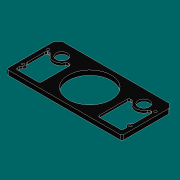
# Autodesk Inventor part: 胴体_メインフレーム_1_2
Saved by Autodesk Inventor 2016 (Build 200138000, 138)
## iProperties
Created: 2016-05-05
Part Number: 胴体_メインフレーム_1_2
Material: アセタール樹脂、黒
Document SubType Name: Modeling
Designer: hiroaki
Density: 1.425 g/cm^3
Appearance: 滑らか - 黒
Mass: 18.1472 g
Surface Area: 107.175 cm^2
Volume: 12.7348 cm^3
Author: hiroaki
Autodesk Inventor part; units mm, degrees
ref_plane "YZ Plane" through (0, 0, 0) normal (1, 0, 0) x (0, 1, 0)
ref_plane "XZ Plane" through (0, 0, 0) normal (0, 1, 0) x (-1, 0, 0)
ref_plane "XY Plane" through (0, 0, 0) normal (0, 0, 1) x (1, 0, 0)
derived "胴体_基礎_1_1.ipt"
sketch "スケッチ1" plane through (0, 0, 0) normal (0, 0, 1) x (1, 0, 0)
  circle A0 centre (44, 0) radius 10.5 construction
  line L0 (0, 0) -> (0, 13.5711) construction
  line L1 (0, 0) -> (44, 0) construction
  line L2 (30.5, -1) -> (57.5, -1) construction
  line L3 (57.5, -1) -> (57.5, -28) construction
  line L4 (57.5, -28) -> (30.5, -28) construction
  line L5 (30.5, -28) -> (30.5, -1) construction
  circle A1 centre (30.5, -1) radius 1.35
  circle A2 centre (57.5, -1) radius 1.35
  circle A3 centre (30.5, -28) radius 1.35
  circle A4 centre (57.5, -28) radius 1.35
  line L6 (28, 0) -> (28, -39.5) construction
  line L7 (28, -39.5) -> (60, -39.5) construction
  line L8 (60, -39.5) -> (60, 0) construction
  line L9 (44, 0) -> (44, -1) construction
  arc A5 (33.417, 12) -> (28, 0) centre (44, 0) ccw construction
  line L10 (33.417, 12) -> (54.583, 12) construction
  arc A6 (60, 0) -> (54.583, 12) centre (44, 0) ccw construction
  circle A7 centre (44, 0) radius 11
  line L11 (56.5, 21.6506) -> (8, -62.3538) construction
  line L12 (31.8157, -76.1038) -> (-15.8157, -48.6038) construction
  line L13 (-15.8157, -48.6038) -> (32.6843, 35.4006) construction
  line L14 (32.6843, 35.4006) -> (80.3157, 7.9006) construction
  line L15 (80.3157, 7.9006) -> (31.8157, -76.1038) construction
  line L16 (-71.5, 25) -> (-16.5, 25) construction
  line L17 (-16.5, 25) -> (-16.5, -72) construction
  line L18 (-16.5, -72) -> (-71.5, -72) construction
  line L19 (-71.5, -72) -> (-71.5, 25) construction
  line L20 (-44, 25) -> (-44, -72) construction
  line L21 (-71.5, 0) -> (-16.5, 0) construction
  line L22 (-52.5, -44.5) -> (52.5, -44.5) construction
  line L23 (52.5, -44.5) -> (52.5, -78) construction
  line L24 (52.5, -78) -> (-52.5, -78) construction
  line L25 (-52.5, -78) -> (-52.5, -44.5) construction
  line L26 (-44.5, -5) -> (44.5, -5) construction
  line L27 (44.5, -5) -> (44.5, -65) construction
  line L28 (44.5, -65) -> (-44.5, -65) construction
  line L29 (-44.5, -65) -> (-44.5, -5) construction
  circle A8 centre (44, 24.25) radius 1.2
  circle A9 centre (19.75, 0) radius 1.2
  circle A10 centre (44, -24.25) radius 1.2
  circle A11 centre (68.25, 0) radius 1.2
  line L30 (-45.0355, 26.75) -> (45.0355, 26.75) construction
  circle A12 centre (44, 24.25) radius 2.5 construction
  line L31 (46, 25.4047) -> (46, 23.0953) construction
  line L32 (46, 23.0953) -> (44, 21.9406) construction
  line L33 (44, 21.9406) -> (42, 23.0953) construction
  line L34 (42, 23.0953) -> (42, 25.4047) construction
  line L35 (42, 25.4047) -> (44, 26.5594) construction
  line L36 (44, 26.5594) -> (46, 25.4047) construction
  line L37 (70.75, 1.0355) -> (70.75, -31.2817) construction
  line L38 (-70.75, -31.2817) -> (-70.75, 1.0355) construction
  circle A13 centre (68.25, 0) radius 2.5 construction
  circle A14 centre (-44, 24.25) radius 1.2
  circle A15 centre (-19.75, 0) radius 1.2
  circle A16 centre (-30.5, -1) radius 1.35
  circle A17 centre (-44, 0) radius 11
  circle A18 centre (-57.5, -1) radius 1.35
  circle A19 centre (-44, -24.25) radius 1.2
  circle A20 centre (-30.5, -28) radius 1.35
  circle A21 centre (-57.5, -28) radius 1.35
  circle A22 centre (-68.25, 0) radius 1.2
  line L39 (-45.0355, 26.75) -> (-70.75, 1.0355) construction
  line L40 (45.0355, 26.75) -> (70.75, 1.0355) construction
  line L41 (70.75, 1.0355) -> (70.75, -1.0355)
  line L42 (-70.75, 1.0355) -> (-70.75, -1.0355) construction
  circle A23 centre (44, 0) radius 6.05
  circle A24 centre (-44, 0) radius 6.05
  line L43 (-70.75, -1.0355) -> (-62, -9.7855) construction
  line L44 (-62, -9.7855) -> (-62, -33) construction
  line L45 (-62, -33) -> (62, -33) construction
  line L46 (62, -33) -> (62, -9.7855) construction
  line L47 (62, -9.7855) -> (70.75, -1.0355) construction
  line L48 (57.7855, 14) -> (-57.7855, 14)
  line L49 (-57.7855, 14) -> (-62, 9.7855)
  line L50 (-62, 9.7855) -> (-62, -41.5)
  line L51 (-62, -41.5) -> (62, -41.5)
  line L52 (62, -41.5) -> (62, 9.7855)
  line L53 (62, 9.7855) -> (57.7855, 14)
  line L54 (21.5, -5) -> (26.5, -5) construction
  line L55 (19.75, 0) -> (28, 0) construction
  circle A25 centre (22.5, -28) radius 1.55 construction
  circle A26 centre (22.5, 21.75) radius 1.55 construction
  circle A27 centre (-22.5, 21.75) radius 1.55 construction
  circle A28 centre (-22.5, -28) radius 1.55 construction
  circle A29 centre (19.75, 0) radius 2 construction
  circle A30 centre (22.5, 21.75) radius 3 construction
  circle A31 centre (-22.5, 21.75) radius 1.2
  circle A32 centre (-22.5, -28) radius 1.2
  circle A33 centre (22.5, 21.75) radius 1.2
  circle A34 centre (22.5, -28) radius 1.2
  line L56 (-25.05, 15.75) -> (-19.95, 15.75) construction
  line L57 (-19.95, 15.75) -> (-19.95, 5.75) construction
  line L58 (-19.95, 5.75) -> (-25.05, 5.75) construction
  line L59 (-25.05, 5.75) -> (-25.05, 15.75) construction
  line L60 (-25.05, -4) -> (-19.95, -4) construction
  line L61 (-19.95, -4) -> (-19.95, -22) construction
  line L62 (-19.95, -22) -> (-25.05, -22) construction
  line L63 (-25.05, -22) -> (-25.05, -4) construction
  circle A35 centre (-19.75, 0) radius 2.5 construction
  line L64 (-19.9, 15.8) -> (-25.1, 15.8)
  line L65 (-25.1, 15.8) -> (-25.1, 5.7)
  line L66 (-25.1, 5.7) -> (-19.9, 5.7)
  line L67 (-19.9, 5.7) -> (-19.9, 15.8)
  circle A36 centre (-25.1, 14.75) radius 1.05
  circle A37 centre (-19.9, 14.75) radius 1.05
  circle A38 centre (-19.9, 6.75) radius 1.05
  circle A39 centre (-25.1, 6.75) radius 1.05
  line L68 (-19.9, -3.95) -> (-25.1, -3.95)
  line L69 (-25.1, -3.95) -> (-25.1, -22.05)
  line L70 (-25.1, -22.05) -> (-19.9, -22.05)
  line L71 (-19.9, -22.05) -> (-19.9, -3.95)
  circle A40 centre (-25.1, -5) radius 1.05
  circle A41 centre (-19.9, -5) radius 1.05
  circle A42 centre (-25.1, -21) radius 1.05
  circle A43 centre (-19.9, -21) radius 1.05
  line L72 (25.1, 15.8) -> (25.1, 5.7)
  circle A44 centre (25.1, 14.75) radius 1.05
  line L73 (19.9, 15.8) -> (25.1, 15.8)
  circle A45 centre (19.9, 14.75) radius 1.05
  line L74 (19.9, 5.7) -> (19.9, 15.8)
  circle A46 centre (25.1, 6.75) radius 1.05
  circle A47 centre (19.9, 6.75) radius 1.05
  line L75 (25.1, 5.7) -> (19.9, 5.7)
  circle A48 centre (25.1, -5) radius 1.05
  circle A49 centre (19.9, -5) radius 1.05
  line L76 (19.9, -3.95) -> (25.1, -3.95)
  line L77 (19.9, -22.05) -> (19.9, -3.95)
  line L78 (25.1, -3.95) -> (25.1, -22.05)
  circle A50 centre (25.1, -21) radius 1.05
  circle A51 centre (19.9, -21) radius 1.05
  line L79 (25.1, -22.05) -> (19.9, -22.05)
  circle A52 centre (44, 0) radius 21.9406 construction
  point P0 (0, -44.5)
  point P1 (-44.5, -35)
  point P2 (0, -5)
  point P3 (-22.5, 15.75)
  point P4 (-22.5, -4)
  point P5 (-22.5, 5.75)
  dimension "d60" = 12.1
  dimension "d61" = 2
  dimension "d64" = 2.4
  dimension "d66" = 14
  measures "d60" diameter of A23
  measures "d61" distance between parallel lines of L51 L7
  measures "d64" diameter of A31
  measures "d66" distance from line of L48 A17.centre
extrude "押し出し1" add sketch "スケッチ1" along normal blind 2.5 contours A1 | A3 | A7 | A9 | A10 | A15 | A16 | A17 | A19 | A20 | L53 L52 L51 L50 L49 L48 A36 L65 A39 L66 A38 L67 A37 A45 L74 A47 L75 A46 L72 A44 | A44 L72 L48 | L72 A44 L48 | L72 A46 L75 A47 L74 A45 L48 A44 | A46 L72 | L72 A46 | A45 L74 L48 | L74 A45 L48 | A47 L74 | L74 A47 | A37 L67 L48 | L48 L65 A36 | L67 A37 L48 | L67 A38 L66 A39 L65 A36 L48 A37 | L48 A36 L65 | A38 L67 | L67 A38 | A39 L65 | L65 A39 | A32 | A34 | A41 L71 A43 L70 A42 L69 A40 L68 | A41 L71 | L71 A41 | A40 L69 | L69 A40 | A43 L71 | L71 A43 | A42 L69 | L69 A42 | A48 L78 | L78 A48 | A48 L78 A50 L79 A51 L77 A49 L76 | L77 A49 | A49 L77 | A50 L78 | L78 A50 | A51 L77 | L77 A51 picked at (25.5372, 13.9575) picked at (24.6628, 13.9575) picked at (20.3372, 13.9575) picked at (19.4628, 13.9575) picked at (-19.4628, 13.9575) picked at (-25.5372, 13.9575) picked at (-20.3372, 13.9575) picked at (-24.6628, 13.9575)
mirror "ミラー1" about plane through (0, -14.1578, 0) normal (0, 0, -1) of "押し出し1"
sketch "スケッチ4" plane through (62, -41.5, -2.5) normal (0, 0, -1) x (-1, 0, 0)
  circle A0 centre (106, 41.5) radius 5.05
  circle A1 centre (4.5, 13.5) radius 1.35 projected
  circle A2 centre (4.5, 40.5) radius 1.35 projected
  circle A3 centre (119.5, 13.5) radius 1.35 projected
  circle A4 centre (119.5, 40.5) radius 1.35 projected
  line L0 (7.417, 53.5) -> (28.583, 53.5) construction
  line L1 (2, 41.5) -> (2, 2) construction
  line L2 (2, 2) -> (34, 2) construction
  line L3 (34, 2) -> (34, 41.5) construction
  arc A5 (7.417, 53.5) -> (2, 41.5) centre (18, 41.5) ccw construction
  arc A6 (34, 41.5) -> (28.583, 53.5) centre (18, 41.5) ccw construction
  line L4 (1.95, 1.95) -> (1.95, 41.5)
  arc A7 (7.3981, 53.55) -> (1.95, 41.5) centre (18, 41.5) ccw
  line L5 (7.3981, 53.55) -> (28.6019, 53.55)
  arc A8 (34.05, 41.5) -> (28.6019, 53.55) centre (18, 41.5) ccw
  line L6 (34.05, 41.5) -> (34.05, 1.95)
  line L7 (34.05, 1.95) -> (1.95, 1.95)
  circle A9 centre (3.3996, 3.3996) radius 2.05
  circle A10 centre (32.6004, 3.3996) radius 2.05
  circle A11 centre (27.7355, 51.6921) radius 2.05
  circle A12 centre (8.2645, 51.6921) radius 2.05
  line L8 (3.3996, 3.3996) -> (1.95, 1.95) construction
  line L9 (8.2645, 51.6921) -> (7.3981, 53.55) construction
  line L10 (62, 41.5) -> (62, 0) construction
  line L11 (122.05, 1.95) -> (122.05, 41.5)
  arc A13 (122.05, 41.5) -> (116.6019, 53.55) centre (106, 41.5) ccw
  line L12 (116.6019, 53.55) -> (95.3981, 53.55)
  arc A14 (95.3981, 53.55) -> (89.95, 41.5) centre (106, 41.5) ccw
  line L13 (89.95, 41.5) -> (89.95, 1.95)
  line L14 (89.95, 1.95) -> (122.05, 1.95)
  circle A15 centre (120.6004, 3.3996) radius 2.05
  circle A16 centre (91.3996, 3.3996) radius 2.05
  circle A17 centre (96.2645, 51.6921) radius 2.05
  circle A18 centre (115.7355, 51.6921) radius 2.05
  circle A19 centre (18, 41.5) radius 5.05
  circle A20 centre (106, 41.5) radius 5.05
  line L15 (124, 0) -> (0, 0) projected
  line L16 (18, 41.5) -> (18, 2) construction
  circle A21 centre (18, 41.5) radius 6.05 projected
  point P0 (18, 53.5)
  point P1 (62, 0)
  dimension "d56" = 4.1
  dimension "d52" = 16
  dimension "d53" = 51.5
  dimension "d54" = 0.05
  dimension "d55" = 45
  dimension "d57" = 65
  dimension "d62" = 10.1
  dimension "d63" = 12
  constraints: 32 end point, 16 symmetric about line, 12 point on circle, 9 centre point, 6 coincident, 6 vertical, 5 perpendicular, 4 midpoint, 2 tangent, 1 equal radius, 1 horizontal, 32 other
  measures "d52" radius of A5
  measures "d53" distance between parallel lines of L2 L0
  measures "d54" distance between parallel lines of L4 L1
  measures "d55" angle of L1 L8
  measures "d57" angle of L0 L9
  measures "d62" diameter of A19
  measures "d63" distance from line of A5.centre L0
extrude "押し出し2" cut sketch "スケッチ4" against normal blind 2.5 contours A9 L4 | L4 A9 L7 | L7 A9 | L4 A7 A12 L5 A11 A8 L6 A10 L7 A9 | A10 L6 L7 | L7 A10 | A12 A7 | A7 L5 A12 | L6 A10 | A12 L5 | A11 L5 A8 | A8 A11 | A11 L5 | L14 A15 L11 | A15 L14 | L11 A15 | A15 L14 A16 L13 A14 A17 L12 A18 A13 L11 | A16 L14 | L14 L13 A16 | A18 L12 A13 | A13 A18 | A16 L13 | L12 A18 | A17 A14 L12 | L12 A17 | A17 A14 | A19 | A21
sketch "スケッチ6" plane through (62, -41.5, -2.5) normal (0, 0, -1) x (-1, 0, 0)
  line L0 (34.05, 41.5) -> (34.05, 4.8491) construction
  line L1 (4.2145, 55.5) -> (119.7855, 55.5) projected
  circle A0 centre (62, 27.55) radius 27.95 construction
  circle A1 centre (62, 27.55) radius 22.95
  line L2 (31.1509, 1.95) -> (4.8491, 1.95) construction
  line L3 (1.95, 4.8491) -> (1.95, 41.5) construction
  arc A2 (6.4482, 52.6426) -> (1.95, 41.5) centre (18, 41.5) ccw construction
  line L4 (4.95, 37.6858) -> (4.95, 16.3142)
  line L5 (4.95, 10.6858) -> (4.95, 4.95)
  line L6 (4.95, 4.95) -> (31.05, 4.95)
  line L7 (31.05, 4.95) -> (31.05, 38.5)
  line L8 (6.5304, 38.5) -> (9.5147, 38.5)
  line L9 (31.05, 38.5) -> (26.4853, 38.5)
  arc A3 (9.5147, 38.5) -> (26.4853, 38.5) centre (18, 41.5) ccw
  arc A4 (4.95, 37.6858) -> (6.5304, 38.5) centre (4.5, 40.5) ccw
  circle A5 centre (4.5, 40.5) radius 1.35 construction
  circle A6 centre (4.5, 40.5) radius 1.35 construction
  arc A7 (4.95, 10.6858) -> (4.95, 16.3142) centre (4.5, 13.5) ccw
  circle A8 centre (4.5, 13.5) radius 1.35 construction
  circle A9 centre (4.5, 13.5) radius 1.35 construction
  line L10 (62, 41.5) -> (62, 27.55) construction
  line L11 (119.05, 37.6858) -> (119.05, 16.3142)
  line L12 (119.05, 10.6858) -> (119.05, 4.95)
  line L13 (119.05, 4.95) -> (92.95, 4.95)
  line L14 (92.95, 4.95) -> (92.95, 38.5)
  line L15 (117.4696, 38.5) -> (114.4853, 38.5)
  line L16 (92.95, 38.5) -> (97.5147, 38.5)
  arc A10 (97.5147, 38.5) -> (114.4853, 38.5) centre (106, 41.5) ccw
  arc A11 (117.4696, 38.5) -> (119.05, 37.6858) centre (119.5, 40.5) ccw
  arc A12 (119.05, 16.3142) -> (119.05, 10.6858) centre (119.5, 13.5) ccw
  arc A13 (1.95, 4.8491) -> (4.8491, 1.95) centre (3.3996, 3.3996) ccw construction
  arc A14 (9.1308, 53.55) -> (6.4482, 52.6426) centre (8.2645, 51.6921) ccw construction
  line L17 (9.1308, 53.55) -> (26.8692, 53.55) construction
  arc A15 (29.5518, 52.6426) -> (26.8692, 53.55) centre (27.7355, 51.6921) ccw construction
  arc A16 (34.05, 41.5) -> (29.5518, 52.6426) centre (18, 41.5) ccw construction
  arc A17 (31.1509, 1.95) -> (34.05, 4.8491) centre (32.6004, 3.3996) ccw construction
  line L18 (124, 0) -> (0, 0) projected
  line L19 (26.8803, 53.5) -> (9.1197, 53.5) construction
  arc A18 (9.1197, 53.5) -> (6.4892, 52.6131) centre (8.2645, 51.6921) ccw construction
  arc A19 (6.4892, 52.6131) -> (2, 41.5) centre (18, 41.5) ccw construction
  line L20 (2, 41.5) -> (2, 4.8283) construction
  arc A20 (2, 4.8283) -> (4.8283, 2) centre (3.3996, 3.3996) ccw construction
  line L21 (4.8283, 2) -> (31.1717, 2) construction
  arc A21 (31.1717, 2) -> (34, 4.8283) centre (32.6004, 3.3996) ccw construction
  line L22 (34, 4.8283) -> (34, 41.5) construction
  arc A22 (34, 41.5) -> (29.5108, 52.6131) centre (18, 41.5) ccw construction
  arc A23 (29.5108, 52.6131) -> (26.8803, 53.5) centre (27.7355, 51.6921) ccw construction
  line L23 (35.3205, 51.5) -> (47.5917, 51.5)
  arc A24 (37.9966, 41.8692) -> (35.3205, 51.5) centre (18, 41.5) ccw
  arc A25 (47.5917, 51.5) -> (37.9966, 41.8692) centre (62, 27.55) ccw
  line L24 (38, 13.2251) -> (38, 4)
  line L25 (38, 4) -> (46.9468, 4)
  arc A26 (38, 13.2251) -> (46.9468, 4) centre (62, 27.55) ccw
  line L26 (88.6795, 51.5) -> (76.4083, 51.5)
  arc A27 (88.6795, 51.5) -> (86.0034, 41.8692) centre (106, 41.5) ccw
  arc A28 (86.0034, 41.8692) -> (76.4083, 51.5) centre (62, 27.55) ccw
  line L27 (86, 13.2251) -> (86, 4)
  line L28 (86, 4) -> (77.0532, 4)
  arc A29 (77.0532, 4) -> (86, 13.2251) centre (62, 27.55) ccw
  dimension "d74" = 5
  dimension "d77" = 9
  dimension "d78" = 1.5
  dimension "d79" = 2
  dimension "d80" = 3
  dimension "d81" = 3
  dimension "d82" = 3
  dimension "d85" = 0.05
  dimension "d89" = 4
  dimension "d90" = 4
  dimension "d91" = 4
  dimension "d92" = 4
  constraints: 46 end point, 36 point on circle, 22 centre point, 19 symmetric about line, 8 coincident, 6 tangent, 4 horizontal, 4 vertical, 2 perpendicular, 2 vertical alignment, 1 equal radius, 1 horizontal alignment, 15 other
  measures "d74" radial gap between concentric circles of A0 A1
  measures "d77" radius of A3
  measures "d78" radial gap between concentric circles of A5 A4
  measures "d79" distance from line of L8 A5.centre
  measures "d80" distance between parallel lines of L3 L4
  measures "d81" distance between parallel lines of L0 L7
  measures "d82" distance between parallel lines of L2 L6
  measures "d85" distance between parallel lines of L17 L19
  measures "d89" radial gap between concentric circles of A24 A22
  measures "d90" distance between parallel lines of L1 L23
  measures "d91" distance between parallel lines of L24 L22
  measures "d92" distance between parallel lines of L18 L25
extrude "押し出し4" cut sketch "スケッチ6" against normal blind 5 contours A1 | A4 L8 A3 L9 L7 L6 L5 A7 L4 | L11 A12 L12 L13 L14 L16 A10 L15 A11
fillet "フィレット2" radius 2 24 edges at (57.05, -36.55, 1.25) (57.05, -30.8142, 1.25) (57.05, -25.1858, 1.25) (57.05, -3.8142, 1.25) (55.4696, -3, 1.25) (52.4853, -3, 1.25) (35.5147, -3, 1.25) (30.95, -3, 1.25) (30.95, -36.55, 1.25) (-30.95, -3, 1.25) (-57.05, -30.8142, 1.25) (-57.05, -36.55, 1.25) (-57.05, -25.1858, 1.25) (-30.95, -36.55, 1.25) (-52.4853, -3, 1.25) (-57.05, -3.8142, 1.25) (-35.5147, -3, 1.25) (-55.4696, -3, 1.25) (-62, -41.5, 0) (-62, 9.7855, 0) (-57.7855, 14, 0) (57.7855, 14, 0) (62, 9.7855, 0) (62, -41.5, 0)
equation "\"d81\" = d80"
equation "\"d82\" = d80"
equation "\"d48\" = 3"
